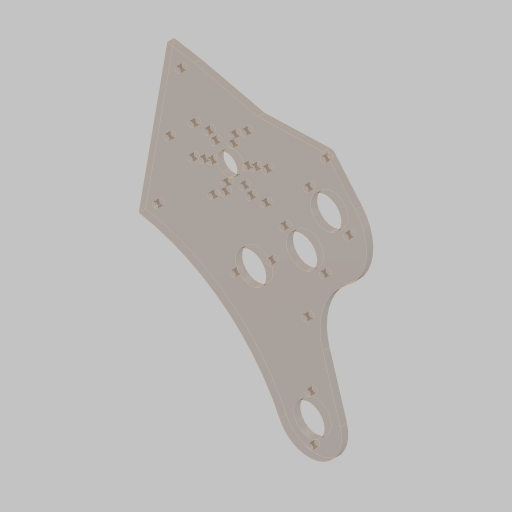
# Autodesk Inventor part: GP10-001
Saved by Autodesk Inventor 2023.5 (Build 275446000, 446)
## iProperties
Created: 2025-02-24
Part Number: GP10-001
Material: Polycarbonate, Smoke
Document SubType Name: Modeling
Designer: dlangdon
Density: 1.2 g/cm^3
Appearance: Polycarbonate - Smoked
Author: dlangdon
Autodesk Inventor part; units mm, degrees
ref_plane "YZ Plane" through (0, 0, 0) normal (1, 0, 0) x (0, 1, 0)
ref_plane "XZ Plane" through (0, 0, 0) normal (0, 1, 0) x (-1, 0, 0)
ref_plane "XY Plane" through (0, 0, 0) normal (0, 0, 1) x (1, 0, 0)
sketch "Sketch1" plane through (0, 0, 0) normal (0, 0, 1) x (1, 0, 0)
  circle A0 centre (71.842, 71.842) radius 50.8 construction
  circle A1 centre (-71.842, -71.842) radius 50.8 construction
  circle A2 centre (0, 0) radius 50.8 construction
  line L0 (-35.921, -35.921) -> (35.921, 35.921) construction
  line L1 (71.842, 71.842) -> (-71.842, -71.842) construction
  line L2 (-4.3707, 6.2419) -> (-4.3707, 50.6116) construction
  line L3 (-226.8798, -122.642) -> (638.5123, -122.642) construction
  circle A3 centre (147.8406, -65.492) radius 57.15 construction
  circle A4 centre (71.842, 71.842) radius 14.2621
  circle A5 centre (-71.842, -71.842) radius 14.2621
  circle A6 centre (-4.3707, 6.2419) radius 57.15 construction
  circle A7 centre (-71.842, -71.842) radius 30.1371 construction
  circle A8 centre (71.842, 71.842) radius 30.1371 construction
  circle A9 centre (-56.3286, 101.6778) radius 14.2621
  line L4 (-56.3286, 101.6778) -> (71.842, 71.842) construction
  circle A10 centre (71.842, 71.842) radius 14.3256 construction
  circle A11 centre (-71.842, -71.842) radius 14.3256 construction
  circle A12 centre (-78.675, 59.5778) radius 14.2621
  line L5 (-71.842, -71.842) -> (-78.675, 59.5778) construction
  circle A13 centre (-78.675, 59.5778) radius 23.8316 construction
  circle A14 centre (-56.3286, 101.6778) radius 23.8316 construction
  line L6 (14.7165, 60.1103) -> (61.7767, 43.4355)
  line L7 (-43.0113, -63.0652) -> (-59.0434, -10.4018)
  arc A15 (14.7165, 60.1103) -> (-59.0434, -10.4018) centre (-4.3707, 6.2419) ccw
  line L8 (-202.9564, 165.4321) -> (-177.9423, 161.0215)
  line L9 (-177.9423, 161.0215) -> (-204.4062, 10.9368) construction
  line L10 (-204.4062, 10.9368) -> (-229.4204, 15.3474) construction
  line L11 (-229.4204, 15.3474) -> (-202.9564, 165.4321) construction
  line L12 (-248.4004, -92.2937) -> (35.0702, -142.2772) construction
  line L13 (-201.8537, 171.6857) -> (161.0026, 107.7043) construction
  line L14 (-201.8537, 171.6857) -> (-248.4004, -92.2937) construction
  circle A16 centre (-147.7392, 94.6182) radius 31.75 construction
  line L15 (-77.4376, 35.7784) -> (-74.4797, -21.1106) construction
  circle A17 centre (13.0879, 85.5189) radius 9.525 construction
  line L16 (-190.4493, 163.2268) -> (-216.9133, 13.1421) construction
  line L17 (-193.206, 147.593) -> (-214.1566, 28.7759) construction
  circle A18 centre (-147.7392, 94.6182) radius 17.4625 construction
  circle A19 centre (-147.7392, 94.6182) radius 9.525
  circle A20 centre (-56.3286, 101.6778) radius 30.1816 construction
  line L18 (-202.9564, 165.4321) -> (-229.4204, 15.3474)
  arc A21 (61.7767, 43.4355) -> (78.6846, 101.1921) centre (71.842, 71.842) ccw
  arc A22 (-99.1524, -84.5852) -> (-43.0113, -63.0652) centre (-71.842, -71.842) ccw
  line L19 (-147.7392, 94.6182) -> (-131.3298, 100.5908) construction
  line L20 (-113.4287, 107.1063) -> (-182.0497, 82.1302) construction
  circle A23 centre (-182.0497, 82.1302) radius 4.7625 construction
  line L21 (0, 0) -> (-4.3707, 6.2419) construction
  circle A24 centre (71.842, 71.842) radius 28.6512 construction
  line L22 (62.334, 44.8145) -> (-61.0615, 88.2239) construction
  line L23 (75.2477, 100.2901) -> (-54.6333, 115.8388) construction
  line L24 (-177.9423, 161.0215) -> (78.6846, 101.1921)
  line L25 (-147.7392, 94.6182) -> (-125.7265, 22.8485) construction
  circle A25 centre (-125.7265, 22.8485) radius 31.75 construction
  circle A26 centre (-125.7265, 22.8485) radius 14.2621
  line L26 (-78.675, 59.5778) -> (-125.7265, 22.8485) construction
  circle A27 centre (-147.7392, 94.6182) radius 25.4 construction
  arc A28 (-99.1524, -84.5852) -> (-229.4204, 15.3474) centre (-260.2996, -159.7777) ccw
  circle A29 centre (-147.7392, 94.6182) radius 36.5125 construction
  line L27 (-180.8308, 110.0491) -> (-147.7392, 94.6182) construction
  arc A30 (-41.9551, 128.217) -> (-49.6289, 131.1064) centre (-56.3286, 101.6778) ccw
  arc A31 (-37.4192, 52.8672) -> (-41.9551, 128.217) centre (-63.1237, 89.1313) ccw
  point P0 (-75.9587, 7.3339)
  point P1 (-203.6813, 88.1845)
  point P2 (-203.6813, 88.1845)
  point P3 (-144.7069, 111.8154)
  point P4 (-161.1163, 105.8429)
  point P5 (-164.1486, 88.6457)
  point P6 (-150.7715, 77.421)
  point P7 (-134.3622, 83.3936)
  point P8 (-123.871, 103.3056)
  point P9 (-143.3285, 119.6324)
  point P10 (-167.1967, 110.945)
  point P11 (-171.6074, 85.9309)
  point P12 (-152.1499, 69.6041)
  point P13 (-128.2817, 78.2914)
  point P14 (-160.2272, 128.9288)
  point P15 (-182.0497, 82.1302)
  point P16 (-135.2512, 60.3077)
  point P17 (-132.3084, 127.7098)
  point P18 (-163.1701, 61.5267)
  point P19 (-114.6476, 79.1874)
  point P20 (-49.4759, 131.0711)
  dimension "d7" = 101.6
  dimension "d18" = 47.6631
  dimension "d34" = 34.925
  dimension "d65" = 50.8
  dimension "d3" = 45
  dimension "d4" = 0
  dimension "d8" = 101.6
  dimension "d9" = 28.5242
  dimension "d10" = 101.6
  dimension "d11" = 114.3
  dimension "d12" = 114.3
  dimension "d13" = 15.875
  dimension "d14" = 15.875
  dimension "d15" = 131.5974
  dimension "d16" = 28.6512
  dimension "d17" = 131.5974
  dimension "d19" = 47.6631
  dimension "d22" = 25.4
  dimension "d23" = 152.4
  dimension "d26" = 268.0517
  dimension "d27" = 63.5
  dimension "d30" = 203.2
  dimension "d31" = 10
  dimension "d32" = 19.05
  dimension "d33" = 120.65
  dimension "d35" = 19.05
  dimension "d36" = 6.35
  dimension "d40" = 360
  dimension "d44" = 9.525
  dimension "d55" = 80
  dimension "d56" = 7.62
  dimension "d57" = 6.35
  dimension "d58" = 57.3024
  dimension "d59" = 63.5
  dimension "d60" = 75.0697
  dimension "d61" = 59.69
  dimension "d62" = 55
  dimension "d68" = 360
  dimension "d70" = 41.275
  dimension "d71" = 60
  dimension "d82" = 360
  dimension "d87" = 360
  dimension "d89" = 45
  dimension "d122" = 44.45
  constraints: 56 end point, 28 point on circle, 27 centre point, 25 coincident, 16 tangent, 7 midpoint, 6 equal radius, 5 point on line, 4 collinear, 4 parallel, 2 horizontal, 1 concentric, 1 perpendicular, 1 vertical, 44 other
  measures "d3" angle of L2 L0
  measures "d4" distance between parallel lines of L0 L1
  measures "d8" diameter of A2
  measures "d9" diameter of A4
  measures "d10" diameter of A0
  measures "d11" diameter of A3
  measures "d12" diameter of A6
  measures "d13" radial gap between concentric circles of A5 A7
  measures "d14" radial gap between concentric circles of A4 A8
  measures "d15" distance of L4.start L4.end
  measures "d16" diameter of A10
  measures "d17" distance of L5.start L5.end
  measures "d19" diameter of A14
  measures "d22" distance of L9.end L10.end
  measures "d23" distance of L10.end L8.start
  measures "d26" distance of L13.start L12.start
  measures "d27" diameter of A16
  measures "d30" distance from line of point (0, 0) L9
  measures "d31" angle of L3 L12
  measures "d32" diameter of A17
  measures "d33" distance of L17.start L17.end
  measures "d35" diameter of A19
  measures "d44" diameter of A23
  measures "d55" angle of L1 L21
  measures "d56" distance of L21.start L21.end
  measures "d57" distance between parallel lines of L13 L8
  measures "d58" diameter of A24
  measures "d59" diameter of A25
  measures "d60" distance of L19.start L25.end
  measures "d61" distance of L26.start L26.end
  measures "d62" angle of L15 L26
  measures "d70" distance from line of L9 L19.start
  measures "d71" angle of L9 L20
  measures "d89" angle of L20 L27
  measures "d122" radius of A31
extrude "Extrusion1" add sketch "Sketch1" along normal blind 6.35 contours A30 A31 A15 L7 A22 A28 L18 L8 L24
hole "Hole1" at (13.0879, 85.5189, 0) at (-193.206, 147.593, 0) at (-203.6813, 88.1845, 0) at (-214.1566, 28.7759, 0) at (-131.3298, 100.5908, 0) at (-144.7069, 111.8154, 0) at (-161.1163, 105.8429, 0) at (-164.1486, 88.6457, 0) at (-150.7715, 77.421, 0) at (-134.3622, 83.3936, 0) at (-113.4287, 107.1063, 0) at (-182.0497, 82.1302, 0) at (-152.1499, 69.6041, 0) at (-171.6074, 85.9309, 0) at (-167.1967, 110.945, 0) at (-143.3285, 119.6324, 0) at (-123.871, 103.3056, 0) at (-128.2817, 78.2914, 0) at (-75.9587, 7.3339, 0) at (-180.8308, 110.0491, 0) at (-132.3084, 127.7098, 0) at (-114.6476, 79.1874, 0) at (-163.1701, 61.5267, 0) direction (0, 0, 1) diameter 5.1054 end through all clearance for "Flat Head Machine Screw (82)" size "#10" standard "Ansi Unified Screw Threads"
sketch "Sketch2" plane through (0, 0, 6.35) normal (0, 0, 1) x (1, 0, 0)
  circle A0 centre (-128.2817, 78.2914) radius 2.5527 construction
  circle A1 centre (-143.3285, 119.6324) radius 2.5527 construction
  circle A2 centre (-171.6074, 85.9309) radius 2.5527 construction
  circle A3 centre (-182.0497, 82.1302) radius 2.5527 construction
  circle A4 centre (-134.3622, 83.3936) radius 2.5527 construction
  circle A5 centre (-164.1486, 88.6457) radius 2.5527 construction
  circle A6 centre (-144.7069, 111.8154) radius 2.5527 construction
  circle A7 centre (-214.1566, 28.7759) radius 2.5527 construction
  circle A8 centre (-193.206, 147.593) radius 2.5527 construction
  circle A9 centre (-203.6813, 88.1845) radius 2.5527 construction
  circle A10 centre (-131.3298, 100.5908) radius 2.5527 construction
  circle A11 centre (-161.1163, 105.8429) radius 2.5527 construction
  circle A12 centre (-150.7715, 77.421) radius 2.5527 construction
  circle A13 centre (-113.4287, 107.1063) radius 2.5527 construction
  circle A14 centre (-152.1499, 69.6041) radius 2.5527 construction
  circle A15 centre (-167.1967, 110.945) radius 2.5527 construction
  circle A16 centre (-123.871, 103.3056) radius 2.5527 construction
  circle A17 centre (-75.9587, 7.3339) radius 2.5527 construction
  line L0 (-43.0113, -63.0652) -> (-59.0434, -10.4018) construction
  arc A18 (-37.4192, 52.8672) -> (-59.0434, -10.4018) centre (-4.3707, 6.2419) ccw construction
  line L1 (-49.4759, 131.0711) -> (-177.9423, 161.0215) construction
  line L2 (-177.9423, 161.0215) -> (-202.9564, 165.4321) construction
  line L3 (-202.9564, 165.4321) -> (-229.4204, 15.3474) construction
  arc A19 (-99.1524, -84.5852) -> (-229.4204, 15.3474) centre (-260.2996, -159.7777) ccw construction
  arc A20 (-99.1524, -84.5852) -> (-43.0113, -63.0652) centre (-71.842, -71.842) ccw construction
  circle A21 centre (-78.675, 59.5778) radius 14.2621 construction
  circle A22 centre (-147.7392, 94.6182) radius 9.525 construction
  circle A23 centre (-125.7265, 22.8485) radius 14.2621 construction
  circle A24 centre (-56.3286, 101.6778) radius 14.2621 construction
  circle A25 centre (-71.842, -71.842) radius 14.2621 construction
  line L4 (-72.9334, -50.8519) -> (-70.7507, -92.8322) construction
  line L5 (-142.2947, 9.915) -> (-109.1584, 35.7819) construction
  line L6 (-97.2403, 69.4322) -> (-60.1097, 49.7235) construction
  line L7 (-74.8938, 111.5322) -> (-37.7633, 91.8235) construction
  line L8 (41.3438, 49.8338) -> (78.4744, 30.1251) construction
  circle A26 centre (-78.675, 59.5778) radius 14.2621 construction
  line L9 (-56.3286, 101.6778) -> (-78.675, 59.5778) construction
  line L10 (-56.3286, 101.6778) -> (59.9091, 39.9795) construction
  line L11 (-78.675, 59.5778) -> (-125.7265, 22.8485) construction
  line L12 (-78.675, 59.5778) -> (-71.842, -71.842) construction
  arc A27 (-37.4192, 52.8672) -> (-41.9551, 128.217) centre (-63.1237, 89.1313) ccw projected
  arc A28 (-41.9551, 128.217) -> (-49.4759, 131.0711) centre (-56.3286, 101.6778) ccw projected
  point P0 (0, 0)
  dimension "d72" = 42.037
  constraints: 19 end point, 13 coincident, 5 midpoint, 4 collinear, 4 equal length, 2 perpendicular
  measures "d72" distance of L4.start L4.end
hole "Hole2" at (-72.9334, -50.8519, 6.35) at (-109.1584, 35.7819, 6.35) at (-70.7507, -92.8322, 6.35) at (-142.2947, 9.915, 6.35) at (-60.1097, 49.7235, 6.35) at (-97.2403, 69.4322, 6.35) at (-37.7633, 91.8235, 6.35) at (-74.8938, 111.5322, 6.35) at (78.4744, 30.1251, 6.35) at (41.3438, 49.8338, 6.35) direction (0, 0, -1) diameter 5.1054 end through all clearance for "Flat Head Machine Screw (82)" size "#10" standard "Ansi Unified Screw Threads"
sketch "Sketch3" plane through (0, 0, 6.35) normal (0, 0, 1) x (1, 0, 0)
  circle A0 centre (-37.7633, 91.8235) radius 2.5527 construction
  circle A1 centre (-60.1097, 49.7235) radius 2.5527 construction
  circle A2 centre (-70.7507, -92.8322) radius 2.5527 construction
  circle A3 centre (-72.9334, -50.8519) radius 2.5527 construction
  circle A4 centre (-109.1584, 35.7819) radius 2.5527 construction
  circle A5 centre (-142.2947, 9.915) radius 2.5527 construction
  circle A6 centre (-97.2403, 69.4322) radius 2.5527 construction
  circle A7 centre (-74.8938, 111.5322) radius 2.5527 construction
  circle A8 centre (-114.6476, 79.1874) radius 2.5527 construction
  circle A9 centre (-180.8308, 110.0491) radius 2.5527 construction
  circle A10 centre (-128.2817, 78.2914) radius 2.5527 construction
  circle A11 centre (-143.3285, 119.6324) radius 2.5527 construction
  circle A12 centre (-171.6074, 85.9309) radius 2.5527 construction
  circle A13 centre (-182.0497, 82.1302) radius 2.5527 construction
  circle A14 centre (-134.3622, 83.3936) radius 2.5527 construction
  circle A15 centre (-164.1486, 88.6457) radius 2.5527 construction
  circle A16 centre (-144.7069, 111.8154) radius 2.5527 construction
  circle A17 centre (-214.1566, 28.7759) radius 2.5527 construction
  circle A18 centre (-193.206, 147.593) radius 2.5527 construction
  circle A19 centre (-203.6813, 88.1845) radius 2.5527 construction
  circle A20 centre (-131.3298, 100.5908) radius 2.5527 construction
  circle A21 centre (-161.1163, 105.8429) radius 2.5527 construction
  circle A22 centre (-150.7715, 77.421) radius 2.5527 construction
  circle A23 centre (-113.4287, 107.1063) radius 2.5527 construction
  circle A24 centre (-152.1499, 69.6041) radius 2.5527 construction
  circle A25 centre (-167.1967, 110.945) radius 2.5527 construction
  circle A26 centre (-123.871, 103.3056) radius 2.5527 construction
  circle A27 centre (-75.9587, 7.3339) radius 2.5527 construction
  circle A28 centre (-132.3084, 127.7098) radius 2.5527 construction
  circle A29 centre (-163.1701, 61.5267) radius 2.5527 construction
  arc A30 (-37.4192, 52.8672) -> (-59.0434, -10.4018) centre (-4.3707, 6.2419) ccw construction
  arc A31 (-37.4192, 52.8672) -> (-41.9551, 128.217) centre (-63.1237, 89.1313) ccw projected
  arc A32 (-41.9551, 128.217) -> (-49.4759, 131.0711) centre (-56.3286, 101.6778) ccw projected
  line L0 (-49.4759, 131.0711) -> (-177.9423, 161.0215) construction
  line L1 (-177.9423, 161.0215) -> (-202.9564, 165.4321) construction
  line L2 (-202.9564, 165.4321) -> (-229.4204, 15.3474) construction
  arc A33 (-99.1524, -84.5852) -> (-229.4204, 15.3474) centre (-260.2996, -159.7777) ccw construction
  arc A34 (-99.1524, -84.5852) -> (-43.0113, -63.0652) centre (-71.842, -71.842) ccw construction
  line L3 (-43.0113, -63.0652) -> (-59.0434, -10.4018) construction
  circle A35 centre (-78.675, 59.5778) radius 14.2621 construction
  circle A36 centre (-125.7265, 22.8485) radius 14.2621 construction
  circle A37 centre (-147.7392, 94.6182) radius 9.525 construction
  circle A38 centre (-56.3286, 101.6778) radius 14.2621 construction
  circle A39 centre (-71.842, -71.842) radius 14.2621 construction
  circle A40 centre (71.832, 71.7988) radius 50.8 construction
  circle A41 centre (71.832, 71.7988) radius 14.2875 construction
  circle A42 centre (71.832, 71.7988) radius 30.1625 construction
  line L4 (-56.3286, 101.6778) -> (71.832, 71.7988) construction
  circle A43 centre (-58.612, 142.9815) radius 69.85 construction
  circle A44 centre (-58.612, 142.9815) radius 101.6 construction
  line L5 (-56.3286, 101.6778) -> (54.8213, 172.1305) construction
  circle A45 centre (54.8213, 172.1305) radius 50.8 construction
  circle A46 centre (54.8213, 172.1305) radius 14.2875 construction
  circle A47 centre (54.8213, 172.1305) radius 30.1625 construction
  circle A48 centre (180.8401, -48.1609) radius 202.9894 construction
  arc A49 (-99.1524, -84.5852) -> (-43.0113, -63.0652) centre (-71.842, -71.842) ccw construction
  circle A50 centre (-71.842, -71.842) radius 50.8 construction
  line L6 (64.454, 101.045) -> (-44.9511, 126.5515) construction
  line L7 (38.6733, 197.6064) -> (-18.1122, 161.6127) construction
  line L8 (39.5139, 116.6399) -> (37.3512, 107.3637) construction
  line L9 (3.4905, 175.3056) -> (-1.6088, 183.3506) construction
  line L10 (39.5139, 116.6399) -> (30.0889, 81.5306) construction
  line L11 (30.0889, 81.5306) -> (71.832, 71.7988) construction
  arc A51 (-52.4278, 141.5398) -> (-58.8199, 149.3281) centre (-58.612, 142.9815) ccw
  line L12 (-49.4759, 131.0711) -> (-177.9423, 161.0215) construction
  line L13 (-58.8199, 149.3281) -> (-119.2878, 147.3469)
  line L14 (-119.2878, 147.3469) -> (-49.4759, 131.0711)
  arc A52 (-37.4192, 52.8672) -> (-41.9551, 128.217) centre (-63.1237, 89.1313) ccw construction
  line L15 (-29.095, 117.7295) -> (-53.7507, 147.067)
  point P0 (0, 0)
  point P1 (31.3192, 81.2438)
  point P2 (-29.095, 117.7295)
  dimension "d95" = 139.7
  dimension "d96" = 203.2
  dimension "d90" = 101.6
  dimension "d91" = 28.575
  dimension "d92" = 15.875
  dimension "d93" = 131.5974
  dimension "d94" = 0
  dimension "d99" = 45.492
  dimension "d100" = 405.9788
  dimension "d101" = 101.6
  dimension "d102" = 9.525
  dimension "d103" = 146.05
  dimension "d104" = 9.525
  dimension "d105" = 41.6552
  dimension "d106" = 41.6552
  dimension "d108" = 42.8625
  dimension "d109" = 9.525
  dimension "d110" = 36.3323
  dimension "d111" = 12.7
  dimension "d112" = 15
  constraints: 22 end point, 8 coincident, 7 centre point, 5 point on circle, 5 point on line, 5 tangent, 3 equal radius, 2 collinear, 2 equal length, 2 parallel, 2 perpendicular, 14 other
  measures "d90" diameter of A40
  measures "d91" diameter of A41
  measures "d93" distance of L4.start L4.end
  measures "d94" angle of L4 L0
  measures "d99" angle of L4 L5
  measures "d100" diameter of A48
  measures "d101" diameter of A50
  measures "d102" distance from line of point (-58.612, 142.982) L0
  measures "d103" distance from line of L2 point (-58.612, 142.982)
  measures "d104" distance of L8.start L8.end
  measures "d105" distance from line of A45.centre L9
  measures "d106" distance from line of L4.end L8
  measures "d108" distance of A40.centre L10.end
  measures "d109" distance of L9.start L9.end
  measures "d110" distance from line of L4 L8.start
  measures "d111" diameter of A51
  measures "d112" angle of L12 L13
extrude "Extrusion2" add sketch "Sketch3" against normal up to surface (6.35 mm away)
sketch "Sketch4" plane through (0, 0, 6.35) normal (0, 0, 1) x (1, 0, 0)
  arc A0 (-53.7507, 147.067) -> (-58.8199, 149.3281) centre (-58.612, 142.9815) ccw construction
  point P0 (0, 0)
  point P1 (-52.4278, 141.5398)
  constraints: 1 coincident
hole "Hole3" at (-58.612, 142.9815, 6.35) direction (0, 0, -1) diameter 5.1054 end through all clearance for "Flat Head Machine Screw (82)" size "#10" standard "Ansi Unified Screw Threads"
body "Solid1"
